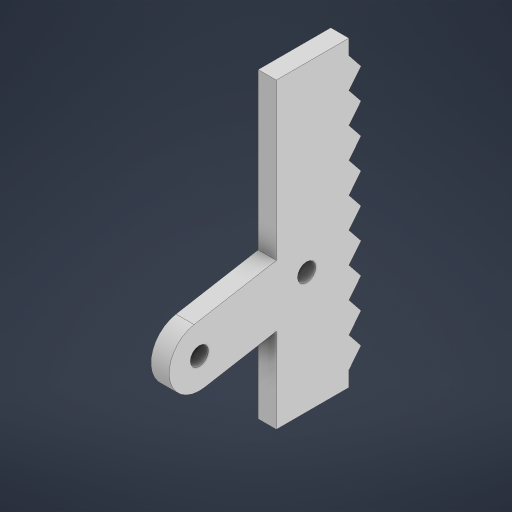
# Autodesk Inventor part: agarre_izquierda
Saved by Autodesk Inventor 2023.1 (Build 271208000, 208)
## iProperties
Created: 2022-10-20
Part Number: agarre_izquierda
Material: Generic
Document SubType Name: Modeling
Designer: amtat
Density: 1 g/cm^3
Appearance: Default
Author: amtat
Autodesk Inventor part; units mm, degrees
ref_plane "YZ Plane" through (0, 0, 0) normal (1, 0, 0) x (0, 1, 0)
ref_plane "XZ Plane" through (0, 0, 0) normal (0, 1, 0) x (-1, 0, 0)
ref_plane "XY Plane" through (0, 0, 0) normal (0, 0, 1) x (1, 0, 0)
sketch "Sketch1" plane through (0, 0, 0) normal (1, 0, 0) x (0, 1, 0)
  line L0 (0, 0) -> (50, 0)
  line L1 (50, 0) -> (20, 0)
  line L2 (20, 0) -> (20, -5)
  circle A0 centre (20, -5) radius 1.5
  line L3 (20, -5) -> (38, -5) construction
  circle A1 centre (16.8743, 12.7265) radius 1.5
  arc A2 (17.7426, 7.8025) -> (11.9503, 11.8583) centre (16.8743, 12.7265) ccw
  line L4 (16.8743, 12.7265) -> (18.3515, 12.987)
  line L5 (16.8743, 12.7265) -> (15.3971, 12.4661)
  line L6 (20, -5) -> (24.924, -4.1318)
  line L7 (24.924, -4.1318) -> (21.7984, 13.5948)
  line L8 (20, -5) -> (15.076, -5.8682)
  line L9 (15.076, -5.8682) -> (11.9503, 11.8583)
  line L10 (20, -5) -> (19.1184, 0)
  line L11 (17.1348, 11.2493) -> (16.8743, 12.7265)
  line L12 (0, 0) -> (0, -12)
  line L13 (50, -12) -> (50, 0)
  line L14 (50, -12) -> (47.5, -12)
  line L15 (45, -12) -> (42.5, -12)
  line L16 (42.5, -12) -> (37.5, -12)
  line L17 (37.5, -12) -> (32.5, -12)
  line L18 (32.5, -12) -> (27.5, -12)
  line L19 (27.5, -12) -> (22.5, -12)
  line L20 (22.5, -12) -> (17.5, -12)
  line L21 (17.5, -12) -> (12.5, -12)
  line L22 (12.5, -12) -> (7.5, -12)
  line L23 (7.5, -12) -> (2.5, -12)
  line L24 (47.5, -12) -> (45, -12)
  line L25 (45, -12) -> (45, -15)
  line L26 (45, -15) -> (47.5, -12)
  line L27 (45, -15) -> (42.5, -12)
  line L28 (42.5, -12) -> (40, -12)
  line L29 (40, -12) -> (40, -15)
  line L30 (40, -15) -> (42.5, -12)
  line L31 (40, -15) -> (37.5, -12)
  line L32 (37.5, -12) -> (35, -12)
  line L33 (35, -12) -> (35, -15)
  line L34 (35, -15) -> (37.5, -12)
  line L35 (35, -15) -> (32.5, -12)
  line L36 (32.5, -12) -> (30, -12)
  line L37 (30, -12) -> (30, -15)
  line L38 (30, -15) -> (32.5, -12)
  line L39 (30, -15) -> (27.5, -12)
  line L40 (27.5, -12) -> (25, -12)
  line L41 (25, -12) -> (25, -15)
  line L42 (25, -15) -> (27.5, -12)
  line L43 (25, -15) -> (22.5, -12)
  line L44 (22.5, -12) -> (20, -12)
  line L45 (20, -12) -> (20, -15)
  line L46 (20, -15) -> (22.5, -12)
  line L47 (20, -15) -> (17.5, -12)
  line L48 (17.5, -12) -> (15, -12)
  line L49 (15, -12) -> (15, -15)
  line L50 (15, -15) -> (17.5, -12)
  line L51 (15, -15) -> (12.5, -12)
  line L52 (12.5, -12) -> (10, -12)
  line L53 (10, -12) -> (10, -15)
  line L54 (10, -15) -> (12.5, -12)
  line L55 (10, -15) -> (7.5, -12)
  line L56 (7.5, -12) -> (5, -12)
  line L57 (5, -12) -> (5, -15)
  line L58 (5, -15) -> (7.5, -12)
  line L59 (5, -15) -> (2.5, -12)
  arc A3 (25, -5) -> (24.924, -4.1318) centre (20, -5) ccw
  arc A4 (20, 0) -> (19.1318, -0.076) centre (20, -5) ccw
  line L60 (0, -12) -> (37.5, -12)
  line L61 (47.5, -12) -> (50, -12)
  line L62 (47.5, -12) -> (45, -12)
  line L63 (45, -12) -> (45, -14)
  line L64 (45, -14) -> (47.5, -12)
  line L65 (45, -14) -> (42.5, -12)
  line L66 (42.5, -12) -> (42.5, -16)
  line L67 (40, -14) -> (37.5, -12)
  line L68 (40, -14) -> (42.5, -12)
  line L69 (37.5, -12) -> (37.5, -16)
  line L70 (30, -14) -> (27.5, -12)
  line L71 (30, -14) -> (32.5, -12)
  line L72 (35, -14) -> (37.5, -12)
  line L73 (35, -14) -> (32.5, -12)
  line L74 (27.5, -12) -> (27.5, -16)
  line L75 (10, -14) -> (7.5, -12)
  line L76 (10, -14) -> (12.5, -12)
  line L77 (15, -14) -> (17.5, -12)
  line L78 (15, -14) -> (12.5, -12)
  line L79 (25, -14) -> (27.5, -12)
  line L80 (25, -14) -> (22.5, -12)
  line L81 (20, -14) -> (22.5, -12)
  line L82 (20, -14) -> (17.5, -12)
  line L83 (7.5, -12) -> (7.5, -16)
  line L84 (5, -14) -> (7.5, -12)
  line L85 (5, -14) -> (2.5, -12)
  point P0 (24.1955, 0)
  point P1 (14.0412, 0)
  point P2 (24.1955, 0)
  point P3 (21.7984, 13.5948)
  dimension "d0" = 50
  dimension "d1" = 30
  dimension "d2" = 5
  dimension "d3" = 3
  dimension "d4" = 18
  dimension "d6" = 3
  dimension "d7" = 10
  dimension "d9" = 5
  dimension "d10" = 12
  dimension "d11" = 100
  dimension "d12" = 2.5
  dimension "d13" = 5
  dimension "d14" = 5
  dimension "d15" = 5
  dimension "d16" = 5
  dimension "d17" = 5
  dimension "d18" = 5
  dimension "d19" = 5
  dimension "d20" = 5
  dimension "d21" = 5
  dimension "d22" = 2.5
  dimension "d23" = 3
  dimension "d24" = 2.5
  dimension "d25" = 3
  dimension "d26" = 2.5
  dimension "d27" = 3
  dimension "d28" = 2.5
  dimension "d29" = 3
  dimension "d30" = 2.5
  dimension "d31" = 3
  dimension "d32" = 2.5
  dimension "d33" = 3
  dimension "d34" = 2.5
  dimension "d35" = 3
  dimension "d36" = 2.5
  dimension "d37" = 3
  dimension "d38" = 2.5
  dimension "d39" = 3
  dimension "d42" = 2
  constraints: 170 end point, 16 perpendicular, 11 vertical, 9 point on circle, 9 point on line, 8 midpoint, 8 symmetric about line, 6 coincident, 5 centre point, 2 horizontal, 2 tangent, 1 collinear, 10 other
  measures "d0" distance of L0.start L0.end
  measures "d1" distance of L0.end L1.end
  measures "d2" distance of L1.end L2.end
  measures "d3" diameter of A0
  measures "d4" distance of L3.start L11.end
  measures "d6" diameter of A1
  measures "d7" diameter of A2
  measures "d9" distance of L4.start L7.end
  measures "d10" distance of L0.start L12.end
  measures "d11" angle of L7 L0
  measures "d12" distance of L13.start L14.end
  measures "d13" distance of L15.end L14.end
  measures "d14" distance of L15.end L16.end
  measures "d15" distance of L16.end L17.end
  measures "d16" distance of L17.end L18.end
  measures "d17" distance of L18.end L19.end
  measures "d18" distance of L19.end L20.end
  measures "d19" distance of L20.end L21.end
  measures "d20" distance of L21.end L22.end
  measures "d21" distance of L22.end L23.end
  measures "d22" distance of L15.start L14.end
  measures "d23" distance of L15.start L25.end
  measures "d24" distance of L15.end L28.end
  measures "d25" distance of L28.end L29.end
  measures "d26" distance of L16.end L32.end
  measures "d27" distance of L32.end L33.end
  measures "d28" distance of L17.end L36.end
  measures "d29" distance of L36.end L37.end
  measures "d30" distance of L18.end L40.end
  measures "d31" distance of L40.end L41.end
  measures "d32" distance of L19.end L44.end
  measures "d33" distance of L44.end L45.end
  measures "d34" distance of L20.end L48.end
  measures "d35" distance of L48.end L49.end
  measures "d36" distance of L21.end L52.end
  measures "d37" distance of L52.end L53.end
  measures "d38" distance of L22.end L56.end
  measures "d39" distance of L56.end L57.end
  measures "d42" distance of L15.start L63.end
extrude "Extrusion2" add sketch "Sketch1" along normal blind 3 contours L0 L9 A2 L7 | L10 A0 L8 L9 L0 | L0 A4 L10 | L0 L7 L6 A0 L2 | L2 A0 L10 A4 | L9 L8 A0 L6 L7 L0 L13 L14 L24 L15 L16 L17 L18 L19 L20 L21 L22 L23 L60 L12 | L23 L57 L85 | L64 L25 L24 | L23 L84 L57 | L25 L65 L15 | L22 L53 L75 | L68 L29 L16 | L22 L76 L53 | L29 L67 L16 | L21 L49 L78 | L72 L33 L17 | L21 L77 L49 | L33 L73 L17 | L20 L45 L82 | L71 L37 L18 | L20 L81 L45 | L37 L70 L18 | L19 L41 L80 | L79 L41 L19
body "Solid2"
